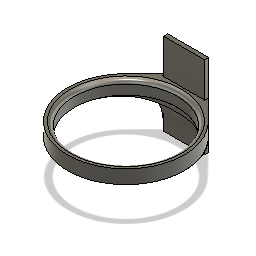
Hair Dryer Stand v4 (Autodesk Fusion 360 design; units mm, degrees)
Autodesk Fusion 360 part; units mm, degrees
sketch "Sketch1" plane through (0, 0, 0) normal (0, 1, 0) x (1, 0, 0) in component "Stand"
  circle A0 centre (0, 0) radius 37.5
  circle A1 centre (0, 0) radius 42.5
  line L0 (-15, 45.5) -> (15, 45.5)
  line L1 (15, 45.5) -> (15, 42.5)
  line L2 (15, 42.5) -> (-15, 42.5)
  line L3 (-15, 42.5) -> (-15, 45.5)
  line L4 (0, 0) -> (0, 45.5) construction
  line L5 (-15, 45.5) -> (-30.4348, 29.6644)
  line L6 (15, 45.5) -> (30.4348, 29.6644)
  dimension "d1" = 75
  dimension "d2" = 85
  dimension "d3" = 3
  dimension "d4" = 30
  constraint coincident A0.centre A1.centre
  constraint horizontal L0
  constraint vertical L1
  constraint horizontal L2
  constraint vertical L3
  constraint tangent A1 L2
  constraint coincident L0 L4.end
  constraint perpendicular L0 L4
  constraint symmetric L1 L3 L4
  constraint coincident A1 L5.end
  constraint tangent A1 L5
  constraint coincident A1 L6.end
  constraint tangent A1 L6
  measures "d1" diameter of A0
  measures "d2" diameter of A1
  measures "d3" distance of L0.end L1.end
  measures "d4" distance of L0.start L0.end
extrude "Extrude1" add sketch "Sketch1" along normal mid plane 10 contours A1 | A1 L1 L2 L6 | A1 L2 L3 L5 makes body 1 in component "Stand"
extrude "Extrude1'" add sketch "Sketch1" along normal mid plane 60 separate body contours L0 L1 L2 L3 makes body 2 in component "Clip"
sketch "Sketch1 (2)" plane through (0, 0, 0) normal (1, 0, 0) x (0, 0, -1) in component "Clip"
  line L0 (42.5, 30) -> (42.5, -30) construction
  line L1 (37.5, -5) -> (-37.5, -5) construction
  spline S0 degree 2 poles (42.5, -30) (42.5, -5) (0, -5) knots 0 0 0 5.982942 5.982942 5.982942 weights 1 3 1
  line L2 (42.5, -30) -> (42.5, -5)
  line L3 (42.5, -5) -> (0, -5)
  constraint coincident L0 L2.end
  constraint midpoint L1 S0.end
  constraint coincident L0.end S0.start
extrude "Extrude2" add sketch "Sketch1 (2)" along normal mid plane 85 bodies 2 in component "Clip"
extrude "Extrude3" cut sketch "Sketch1" against normal blind 50 contours A0 bodies 2 in component "Clip"
sketch "Sketch2" plane through (0, -5, 0) normal (0, 1, 0) x (-1, 0, 0) in component "Clip"
  arc A0 (-37.5, 0) -> (37.5, 0) centre (0, 0) ccw
  line L0 (-37.5, 0) -> (-42.5, 0)
  line L1 (-42.5, 0) -> (-42.5, -42.5)
  line L2 (-42.5, -42.5) -> (-15, -42.5)
  line L3 (-15, -42.5) -> (15, -42.5)
  line L4 (15, -42.5) -> (42.5, -42.5)
  line L5 (42.5, -42.5) -> (42.5, 0)
  line L6 (42.5, 0) -> (37.5, 0)
  circle A1 centre (0, 0) radius 37.5 construction
  line L7 (-15, -42.5) -> (15, -42.5) construction
  line L8 (15, -42.5) -> (15, -45.5) construction
  line L9 (15, -45.5) -> (30.4348, -29.6644) construction
  arc A2 (30.4348, -29.6644) -> (-30.4348, -29.6644) centre (0, 0) ccw construction
  line L10 (-30.4348, -29.6644) -> (-15, -45.5) construction
  line L11 (-15, -45.5) -> (-15, -42.5) construction
  line L12 (42.5, 0) -> (42.5, -42.5)
  line L13 (-42.5, -42.5) -> (-42.5, 0)
  line L14 (-15, -42.5) -> (-26.6769, -33.0846)
  line L15 (15, -42.5) -> (26.6769, -33.0846)
  circle A3 centre (0, 0) radius 42.5
  constraint coincident L5.end L6.start
  constraint coincident L4.end L5.start
  constraint coincident L1.end L2.start
  constraint coincident L0.end L1.start
  constraint coincident L2.end L3.start
  constraint coincident L3.end L4.start
  constraint coincident L15.end A3
  constraint tangent L15 A3
  constraint tangent L14 A3
  constraint coincident L14.end A3
extrude "Extrude4" cut sketch "Sketch2" against normal through all contours L1 L2 L13 L14 A3 | L4 L5 L12 L15 A3 bodies 2 in component "Clip"
fillet "Fillet1" radius 3 1 edges at (-34.9623, 5, -13.5606) on bodies 1 in component "Stand"
move_face "OffsetFaces1" offset -0.5 1 faces at (-5, 1.6667, -42.5) on bodies 1 in component "Stand"
move_face "OffsetFaces2" offset -0.5 1 faces at (15, -1.6667, -44.3333) on bodies 1 in component "Stand"
move_face "OffsetFaces3" offset -0.5 1 faces at (-15, 1.6667, -43.1667) on bodies 1 in component "Stand"
component "Stand" placed x (1, 0, 0) y (0, 1, 0) z (0, 0, 1) at (0, 0, 0)
component "Clip" placed x (1, 0, 0) y (0, 1, 0) z (0, 0, 1) at (0, 0, 0) in component "Stand"
